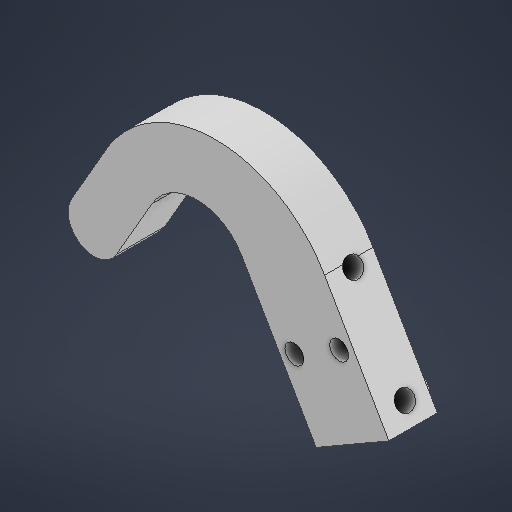
# Autodesk Inventor part: Pass_Hang_Hook
Saved by Autodesk Inventor 2025.1 (Build 291241000, 241)
## iProperties
Created: 2025-01-10
Part Number: Pass_Hang_Hook
Material: Generic
Document SubType Name: Modeling
Designer: Juanl
Density: 1 g/cm^3
Appearance: Default
Author: Juanl
Autodesk Inventor part; units mm, degrees
ref_plane "YZ Plane" through (0, 0, 0) normal (1, 0, 0) x (0, 1, 0)
ref_plane "XZ Plane" through (0, 0, 0) normal (0, 1, 0) x (-1, 0, 0)
ref_plane "XY Plane" through (0, 0, 0) normal (0, 0, 1) x (1, 0, 0)
sketch "Sketch1" plane through (0, 0, 0) normal (0, 0, 1) x (1, 0, 0)
  line L0 (17.67758, 12.244033) -> (26.121491, -2.38125)
  line L1 (10.998523, 23.8125) -> (17.67758, 12.244033)
  arc A0 (15.122969, -21.43125) -> (26.121491, -2.38125) centre (15.122969, -8.73125) ccw
  line L2 (15.122969, -21.43125) -> (-15.122969, -21.43125)
  arc A1 (-26.121491, -2.38125) -> (-15.122969, -21.43125) centre (-15.122969, -8.73125) ccw
  line L3 (-26.121491, -2.38125) -> (-10.998523, 23.8125)
  arc A2 (10.998523, 23.8125) -> (-10.998523, 23.8125) centre (0, 17.4625) ccw
  line L4 (-26.121491, -2.38125) -> (26.121491, -2.38125)
  line L5 (17.90022, 31.333291) -> (26.344131, 16.708008)
  line L6 (11.221163, 42.901758) -> (17.90022, 31.333291)
  line L7 (-19.548851, 27.70653) -> (-10.798548, 42.8625)
  arc A3 (11.221163, 42.901758) -> (-10.798548, 42.8625) centre (0.222593, 36.551839) ccw
  line L8 (26.344131, 16.708008) -> (37.342654, 23.058008)
  line L9 (-30.547374, 34.05653) -> (-21.774405, 49.251758)
  line L10 (37.342654, 23.058008) -> (22.219685, 49.251758)
  arc A4 (22.219685, 49.251758) -> (-21.774405, 49.251758) centre (0.22264, 36.551758) ccw
  arc A5 (26.344131, 16.708008) -> (37.342654, 23.058008) centre (31.843392, 19.883008) ccw
  line L11 (-25.048113, 30.88153) -> (-30.547374, 34.05653)
  line L12 (-30.547374, 34.05653) -> (-19.548851, 27.70653)
  arc A6 (-30.547374, 34.05653) -> (-19.548851, 27.70653) centre (-25.048113, 30.88153) ccw
  line L13 (26.344131, 16.708008) -> (29.519131, 11.208746)
  line L14 (29.519131, 11.208746) -> (40.517654, 17.558746)
  line L15 (40.517654, 17.558746) -> (37.342654, 23.058008)
  point P0 (0, 0)
  point P1 (0, 0)
  point P2 (0, 30.1625)
  point P3 (0.199951, 49.251819)
  point P4 (35.018392, 14.383746)
  dimension "d5" = 12.7
  dimension "d6" = 25.4
  dimension "d7" = 6.35
  dimension "d16" = 6.35
  constraints: 32 end point, 16 point on circle, 7 centre point, 3 horizontal, 2 perpendicular, 2 tangent, 1 parallel, 1 point on line, 14 other
  measures "d5" distance of L5.end L8.end
  measures "d6" radius of A4
  measures "d7" radius of A5
  measures "d16" distance of L5.end L13.end
extrude "Extrusion1" add sketch "Sketch1" along normal blind 11.9126 contours L6 A3 L7 L12 L11 L9 A4 L10 L8 L5 | L8 A5 | A5 L14 L13 | L15 L14 A5 | A6 L11 L12
sketch "Sketch2" plane through (0, 0, 11.9126) normal (0, 0, 1) x (1, 0, 0)
  line L0 (-19.548851, 27.70653) -> (-10.798548, 42.8625)
  arc A0 (11.221163, 42.901758) -> (-10.798548, 42.8625) centre (0.222593, 36.551839) ccw
  arc A1 (22.219685, 49.251758) -> (-21.774405, 49.251758) centre (0.22264, 36.551758) ccw
  line L1 (-21.774405, 49.251758) -> (-30.547374, 34.05653)
  arc A2 (-30.547374, 34.05653) -> (-19.548851, 27.70653) centre (-25.048113, 30.88153) ccw
  line L2 (22.219685, 49.251758) -> (11.221163, 42.901758)
  line L3 (11.221163, 42.901758) -> (29.519131, 11.208746)
  line L4 (29.519131, 11.208746) -> (40.517654, 17.558746)
  line L5 (40.517654, 17.558746) -> (22.219685, 49.251758)
  point P0 (0, 0)
  constraints: 2 end point
sketch "Sketch4" plane through (22.219685, 49.251758, 11.9126) normal (0.8660254, 0.5, 0) x (0, 0, -1)
  line L0 (11.9126, -36.595937) -> (11.9126, 0)
  line L1 (11.9126, 0) -> (0, 0)
  line L2 (0, -36.595937) -> (0, 0)
  line L3 (11.9126, -36.595937) -> (0, -36.595937)
  line L4 (0, 0) -> (6.35, 0)
  line L5 (6.35, 0) -> (6.35, -6.35)
  circle A0 centre (6.35, -6.35) radius 2.3241
  line L6 (6.35, -6.35) -> (6.35, -31.75)
  circle A1 centre (6.35, -31.75) radius 2.3241
  point P0 (11.9126, -31.543431)
  dimension "d17" = 6.35
  dimension "d18" = 6.35
  dimension "d19" = 4.6482
  dimension "d20" = 25.4
  dimension "d21" = 4.6482
  constraints: 6 end point, 2 centre point, 2 coincident, 2 point on line, 1 perpendicular
  measures "d17" distance of L1.end L4.end
  measures "d18" distance of L4.end L5.end
  measures "d19" diameter of A0
  measures "d20" distance of L6.start L6.end
  measures "d21" diameter of A1
extrude "Extrusion2" cut sketch "Sketch4" against normal blind 25.4 contours A0 L6 L5 | L5 L6 A0 | A1
sketch "Sketch5" plane through (0, 0, 0) normal (0, 0, -1) x (-1, 0, 0)
  line L0 (19.548851, 27.70653) -> (10.798548, 42.8625)
  arc A0 (19.548851, 27.70653) -> (30.547374, 34.05653) centre (25.048113, 30.88153) ccw
  line L1 (21.774405, 49.251758) -> (30.547374, 34.05653)
  arc A1 (21.774405, 49.251758) -> (-22.219685, 49.251758) centre (-0.22264, 36.551758) ccw
  line L2 (-40.517654, 17.558746) -> (-22.219685, 49.251758)
  line L3 (-29.519131, 11.208746) -> (-40.517654, 17.558746)
  line L4 (-11.221163, 42.901758) -> (-29.519131, 11.208746)
  arc A2 (10.798548, 42.8625) -> (-11.221163, 42.901758) centre (-0.222593, 36.551839) ccw
  line L5 (-40.517654, 17.558746) -> (-47.402729, 21.533846)
  line L6 (-22.219685, 49.251758) -> (-29.10476, 53.226858)
  line L7 (-29.10476, 53.226858) -> (-47.402729, 21.533846)
  point P0 (0, 0)
  dimension "d24" = 7.9502
  dimension "d25" = 7.9502
  constraints: 6 end point, 1 perpendicular
  measures "d24" distance of L2.start L5.end
  measures "d25" distance of L2.end L6.end
extrude "Extrusion3" add sketch "Sketch5" against normal up to surface (11.9126 mm away) contours L2 L5 L7 L6
sketch "Sketch6" plane through (29.519131, 11.208746, 0) normal (-0.8660254, -0.5, 0) x (0, 0, 1)
  circle A0 centre (5.5626, 30.245937) radius 2.3241
  circle A1 centre (5.5626, 4.845937) radius 2.3241
  line L0 (0, 36.595937) -> (0, 0)
  line L1 (0, 0) -> (11.9126, 0)
  line L2 (11.9126, 36.595937) -> (11.9126, 0)
  line L3 (0, 36.595937) -> (11.9126, 36.595937)
  point P0 (0, 5.052506)
extrude "Extrusion4" cut sketch "Sketch6" against normal through all contours A0 | A1
sketch "Sketch7" plane through (0, 0, 0) normal (0, 0, -1) x (-1, 0, 0)
  line L0 (19.548851, 27.70653) -> (10.798548, 42.8625)
  arc A0 (19.548851, 27.70653) -> (30.547374, 34.05653) centre (25.048113, 30.88153) ccw
  line L1 (21.774405, 49.251758) -> (30.547374, 34.05653)
  arc A1 (21.774405, 49.251758) -> (-22.219685, 49.251758) centre (-0.22264, 36.551758) ccw
  line L2 (-22.219685, 49.251758) -> (-29.10476, 53.226858)
  line L3 (-29.10476, 53.226858) -> (-47.402729, 21.533846)
  line L4 (-29.519131, 11.208746) -> (-47.402729, 21.533846)
  line L5 (-11.221163, 42.901758) -> (-29.519131, 11.208746)
  arc A2 (10.798548, 42.8625) -> (-11.221163, 42.901758) centre (-0.222593, 36.551839) ccw
  line L6 (-29.10476, 53.226858) -> (-8.745927, 60.479014)
  line L7 (-0.22264, 61.951758) -> (-29.10476, 61.951758)
  line L8 (-29.10476, 61.951758) -> (-29.10476, 53.226858)
  arc A3 (-0.22264, 61.951758) -> (-29.10476, 53.226858) centre (-0.22264, 9.784927) ccw
  point P0 (0, 0)
  constraints: 6 end point, 4 point on circle, 2 tangent, 1 centre point, 1 horizontal, 1 perpendicular
extrude "Extrusion5" add sketch "Sketch7" against normal up to surface (11.9126 mm away) contours A1 L6 A3 | A1 L2 L6
fillet "Fillet1" radius 19.05 1 edges at (29.1048, 53.2269, 5.9563)
sketch "Sketch8" plane through (0, 0, 11.9126) normal (0, 0, 1) x (1, 0, 0)
  arc A0 (31.607483, 48.892015) -> (23.673274, 56.383704) centre (15.109699, 39.367015) ccw
  arc A1 (23.673274, 56.383704) -> (0.22264, 61.951758) centre (0.22264, 9.784927) ccw
  arc A2 (0.22264, 61.951758) -> (-21.774405, 49.251758) centre (0.22264, 36.551758) ccw
  line L0 (-21.774405, 49.251758) -> (-30.547374, 34.05653)
  arc A3 (-30.547374, 34.05653) -> (-19.548851, 27.70653) centre (-25.048113, 30.88153) ccw
  line L1 (-19.548851, 27.70653) -> (-10.798548, 42.8625)
  arc A4 (11.221163, 42.901758) -> (-10.798548, 42.8625) centre (0.222593, 36.551839) ccw
  line L2 (11.221163, 42.901758) -> (29.519131, 11.208746)
  line L3 (29.519131, 11.208746) -> (47.402729, 21.533846)
  line L4 (31.607483, 48.892015) -> (47.402729, 21.533846)
  line L5 (31.607483, 48.892015) -> (31.607483, 48.892015)
  line L6 (15.558213, 35.389767) -> (13.234113, 39.415226)
  line L7 (43.81771, 27.743281) -> (46.14181, 23.717822)
  line L8 (28.258213, 13.392722) -> (25.934113, 17.418181)
  line L9 (43.81771, 27.743281) -> (46.14181, 23.717822)
  line L10 (22.219791, 49.251819) -> (31.607483, 54.671805)
  line L11 (31.607483, 48.892015) -> (33.44181, 45.714867)
  line L12 (33.44181, 45.714867) -> (29.10476, 53.226858)
  line L13 (29.10476, 53.226858) -> (32.27976, 47.727596)
  line L14 (32.27976, 47.727596) -> (44.97976, 25.730551)
  line L15 (32.27976, 47.727596) -> (38.62976, 36.729074)
  line L16 (38.62976, 36.729074) -> (29.687961, 31.566524)
  line L17 (29.687961, 31.566524) -> (35.187223, 34.741524)
  circle A5 centre (35.187223, 34.741524) radius 2.3241
  line L18 (35.187223, 34.741524) -> (24.1887, 28.391524)
  circle A6 centre (24.1887, 28.391524) radius 2.3241
  point P0 (0, 0)
  dimension "d33" = 6.35
  dimension "d34" = 25.4
  dimension "d35" = 12.7
  dimension "d36" = 10.3251
  dimension "d52" = 6.35
  dimension "d53" = 4.6482
  dimension "d58" = 12.7
  dimension "d59" = 4.6482
  constraints: 16 end point, 4 point on line, 3 coincident, 2 centre point, 2 midpoint, 1 perpendicular
  measures "d33" distance of L12.end L13.end
  measures "d34" distance of L13.end L14.end
  measures "d35" distance of L13.end L15.end
  measures "d36" distance of L15.end L16.end
  measures "d52" distance of L17.start L17.end
  measures "d53" diameter of A5
  measures "d58" distance of L18.start L18.end
  measures "d59" diameter of A6
extrude "Extrusion6" [suppressed]
sketch "Sketch9" plane through (0, 0, 0) normal (0, 0, -1) x (-1, 0, 0)
  arc A0 (-23.673274, 56.383704) -> (-31.607483, 48.892015) centre (-15.109699, 39.367015) ccw
  line L0 (-31.607483, 48.892015) -> (-47.402729, 21.533846)
  line L1 (-29.519131, 11.208746) -> (-47.402729, 21.533846)
  line L2 (-11.221163, 42.901758) -> (-29.519131, 11.208746)
  arc A1 (10.798548, 42.8625) -> (-11.221163, 42.901758) centre (-0.222593, 36.551839) ccw
  line L3 (19.548851, 27.70653) -> (10.798548, 42.8625)
  arc A2 (19.548851, 27.70653) -> (30.547374, 34.05653) centre (25.048113, 30.88153) ccw
  line L4 (21.774405, 49.251758) -> (30.547374, 34.05653)
  arc A3 (21.774405, 49.251758) -> (-0.22264, 61.951758) centre (-0.22264, 36.551758) ccw
  arc A4 (-0.22264, 61.951758) -> (-23.673274, 56.383704) centre (-0.22264, 9.784927) ccw
  arc A5 (-39.718896, 22.500711) -> (-39.552204, 22.789429) centre (-41.537223, 23.743001) ccw
  arc A6 (-16.020373, 38.147756) -> (-15.931556, 38.288956) centre (-17.8387, 39.390046) ccw
  line L5 (-43.444367, 24.844091) -> (-42.990977, 25.629386)
  line L6 (-40.436133, 25.650145) -> (-41.221427, 26.103535)
  line L7 (-42.638313, 21.835857) -> (-43.423607, 22.289247)
  line L8 (-43.444367, 24.844091) -> (-43.897757, 24.058797)
  line L9 (-43.897757, 24.058797) -> (-42.990977, 25.629386)
  line L10 (-41.221427, 26.103535) -> (-39.65631, 25.199914)
  line L11 (-39.18216, 23.430365) -> (-40.08894, 21.859776)
  line L12 (-41.85849, 21.385626) -> (-43.423607, 22.289247)
  arc A7 (21.774405, 49.251758) -> (-31.607483, 48.892015) centre (-4.811067, 33.421098) ccw
  arc A8 (-43.897757, 24.058797) -> (-43.423607, 22.289247) centre (-42.775907, 23.411097) ccw
  arc A9 (-41.85849, 21.385626) -> (-40.08894, 21.859776) centre (-41.21079, 22.507476) ccw
  arc A10 (-39.18216, 23.430365) -> (-39.65631, 25.199914) centre (-40.30401, 24.078065) ccw
  arc A11 (-41.221427, 26.103535) -> (-42.990977, 25.629386) centre (-41.869127, 24.981686) ccw
  line L13 (-18.93979, 37.482903) -> (-19.725085, 37.936293)
  line L14 (-19.745844, 40.491136) -> (-20.199234, 39.705842)
  line L15 (-18.93979, 37.482903) -> (-18.154496, 37.029513)
  line L16 (-15.937028, 38.292115) -> (-15.931556, 38.288956)
  line L17 (-15.931556, 38.288956) -> (-16.384946, 37.503662)
  line L18 (-19.725085, 37.936293) -> (-18.154496, 37.029513)
  line L19 (-16.384946, 37.503662) -> (-15.478166, 39.074251)
  line L20 (-15.952316, 40.8438) -> (-17.522905, 41.75058)
  line L21 (-19.292454, 41.276431) -> (-20.199234, 39.705842)
  arc A12 (-20.199234, 39.705842) -> (-19.725085, 37.936293) centre (-19.077385, 39.058142) ccw
  arc A13 (-17.522905, 41.75058) -> (-19.292454, 41.276431) centre (-18.170605, 40.628731) ccw
  arc A14 (-15.478166, 39.074251) -> (-15.952316, 40.8438) centre (-16.600016, 39.721951) ccw
  arc A15 (-18.154496, 37.029513) -> (-16.384946, 37.503662) centre (-17.506796, 38.151362) ccw
  point P0 (0, 0)
  point P1 (19.624931, 52.402118)
  dimension "d44" = 1.2954
  dimension "d45" = 1.2954
  constraints: 34 end point, 23 tangent, 22 point on circle, 11 centre point, 8 perpendicular, 6 equal radius, 4 parallel, 4 point on line, 3 midpoint
  measures "d44" radius of A8
  measures "d45" radius of A12
extrude "Extrusion7" add sketch "Sketch9" along normal blind 1.6002 contours L11 A9 L12 L7 A8 L8 L5 A11 L6 L10 A10 | L13 A12 L14 L21 A13 L20 A14 L19 L17 A15 L15
extrude "Extrusion8" add sketch "Sketch9" against normal up to surface (11.9126 mm away) contours A0 A7 A3 A4
sketch "Sketch10" plane through (47.402729, 21.533846, 11.9126) normal (0.8660254, 0.5, 0) x (0, 0, -1)
  line L0 (0, 31.590492) -> (4.454318, 31.590492)
  line L1 (0, 31.590492) -> (0, 0)
  line L2 (11.9126, 0) -> (0, 0)
  line L3 (11.9126, 31.590492) -> (11.9126, 0)
  line L4 (8.245682, 31.590492) -> (11.9126, 31.590492)
  arc A0 (4.454318, 31.590492) -> (8.245682, 31.590492) centre (6.35, 30.245937) ccw
  circle A1 centre (6.35, 4.845937) radius 2.3241
  circle A2 centre (6.35, 30.245937) radius 2.3241
  point P0 (11.9126, 5.052506)
  point P1 (4.454318, 31.590492)
  constraints: 1 centre point, 1 coincident, 1 concentric
extrude "Extrusion9" cut sketch "Sketch10" along normal through all both and the other way through all contours A2 A0
extrude "Extrusion10" cut sketch "Sketch8" against normal through all contours A5 L16 | L16 A5
extrude "Extrusion11" cut sketch "Sketch8" along normal through all both and the other way through all contours A6
body "Solid1"
